Autodesk Inventor part; units mm, degrees
(part 3 of 3)
sketch "Boceto7" plane through (0, 0.45, 0) normal (0, 1, 0) x (1, 0, 0)
  line L0 (-232.1, -160.75) -> (-232.1, 160.75) construction
  line L1 (-232.1, 109.95) -> (232.1, 109.95) construction
  line L2 (232.1, -160.75) -> (232.1, 160.75) construction
  line L3 (-232.1, -109.95) -> (232.1, -109.95) construction
  line L4 (-232.1, 160.75) -> (232.1, 160.75) construction
  line L5 (232.1, -160.75) -> (-232.1, -160.75) construction
  line L6 (232.1, 160.75) -> (-232.1, 160.75) construction
  line L7 (-219.4, 160.75) -> (-219.4, -160.75) construction
  line L8 (-232.1, -160.75) -> (232.1, -160.75) construction
  line L9 (219.4, 160.75) -> (219.4, -160.75) construction
  circle A0 centre (-219.4, 109.95) radius 1.2
  circle A1 centre (219.4, 109.95) radius 1.2
  circle A2 centre (-219.4, -109.95) radius 1.2
  circle A3 centre (219.4, -109.95) radius 1.2
  point P0 (0, 0)
  dimension "d46" = 50.8
  dimension "d47" = 50.8
  dimension "d48" = 12.7
  dimension "d49" = 12.7
  dimension "d50" = 2.4
  dimension "d51" = 2.4
  dimension "d52" = 2.4
  dimension "d53" = 2.4
  constraints: 14 point on line, 8 end point, 4 centre point, 2 horizontal, 2 perpendicular
  measures "d46" distance between parallel lines of L4 L1
  measures "d47" distance between parallel lines of L5 L3
  measures "d48" distance between parallel lines of L0 L7
  measures "d49" distance between parallel lines of L2 L9
  measures "d50" diameter of A0
  measures "d51" diameter of A1
  measures "d52" diameter of A2
  measures "d53" diameter of A3
extrude "Cortar1" cut sketch "Boceto7" against normal blind 0.45
equation "\"d50\" = d51"
equation "\"d52\" = d51"
equation "\"d53\" = d51"
equation "\"d54\" = Grosor"
equation "\"d2\" = Grosor"
equation "\"Radio_pliegue\" = Grosor"
equation "\"Anchura_desahogo_plegado\" = Grosor"
equation "\"Profundidad_desahogo_plegado\" = 0.5 * Grosor"
equation "\"Tamaño_destalonado\" = 4 * Grosor"
equation "\"Remanente_mínimo\" = 2 * Grosor"
equation "\"Radiodetransición\" = Radio_pliegue"
equation "\"Tamaño_de_radio_de_Jacobi\" = Radio_pliegue"
equation "\"TamañoSeparación\" = Grosor"
equation "\"Grosor\" = 0.45"
